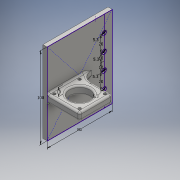
# Autodesk Inventor part: Motor pulley holder
Saved by Autodesk Inventor 2016 (Build 200138000, 138)
## iProperties
Created: 2016-03-20
Part Number: Motor pulley holder
Material: Generic
Document SubType Name: Modeling
Designer: Solomon
Density: 1 g/cm^3
Appearance: Default
Author: Solomon
Autodesk Inventor part; units mm, degrees
ref_plane "YZ Plane" through (0, 0, 0) normal (1, 0, 0) x (0, 1, 0)
ref_plane "XZ Plane" through (0, 0, 0) normal (0, 1, 0) x (-1, 0, 0)
ref_plane "XY Plane" through (0, 0, 0) normal (0, 0, 1) x (1, 0, 0)
sketch "Sketch2" plane through (0, 0, 0) normal (1, 0, 0) x (0, 1, 0)
  line L0 (40, 50) -> (-40, 50)
  line L1 (-40, 50) -> (-40, -50)
  line L2 (-40, -50) -> (40, -50)
  line L3 (40, -50) -> (40, 50)
  line L4 (40, 50) -> (-40, -50) construction
  line L5 (-40, 50) -> (40, -50) construction
  line L6 (40, 50) -> (0, 50)
  line L7 (20, 50) -> (40, 50)
  line L8 (30, 50) -> (30, -50)
  line L9 (30, 0) -> (30, -10)
  line L10 (30, 0) -> (30, 10)
  line L11 (30, -10) -> (30, -30)
  line L12 (30, 10) -> (30, 11.3119)
  line L13 (30, 10) -> (30, 30)
  circle A0 centre (30, -10) radius 2.65
  circle A1 centre (30, 10) radius 2.65
  circle A2 centre (30, 30) radius 2.65
  circle A3 centre (30, -30) radius 2.65
  line L14 (0, 0) -> (-40, 0)
  line L15 (-20, 0) -> (-20, -10)
  line L16 (0, 0) -> (-40, 0)
  line L17 (-40, 0) -> (-40, -10)
  line L18 (-40, -10) -> (0, -10)
  line L19 (0, -10) -> (0, 0)
  line L20 (0, 0) -> (-40, -10) construction
  line L21 (-40, 0) -> (0, -10) construction
  point P0 (-20, -5)
  dimension "d12" = 80
  dimension "d13" = 100
  dimension "d14" = 10
  dimension "d15" = 10
  dimension "d16" = 20
  dimension "d17" = 20
  dimension "d18" = 5.3
  dimension "d19" = 5.3
  dimension "d20" = 5.3
  dimension "d21" = 5.3
  dimension "d22" = 10
  constraints: 44 end point, 11 midpoint, 7 point on line, 4 centre point, 4 coincident, 4 parallel, 3 perpendicular, 2 horizontal, 1 collinear, 1 vertical
  measures "d12" distance of L2.end L1.end
  measures "d13" distance of L1.end L0.end
  measures "d14" distance of L9.start L9.end
  measures "d15" distance of L9.start L10.end
  measures "d16" distance of L9.end L11.end
  measures "d17" distance of L10.end L13.end
  measures "d18" diameter of A0
  measures "d19" diameter of A1
  measures "d20" diameter of A2
  measures "d21" diameter of A3
  measures "d22" distance of L15.start L15.end
extrude "Extrusion2" add sketch "Sketch2" against normal blind 5 contours L3 L2 L8 A3 A0 A1 A2 L0 | L8 A2 A1 A0 A3 L2 L1 L18 L19 L14 L0 | A2 L8 | L8 A2 | A3 L8 | L8 A3 | A1 L8 | L8 A1 | A0 L8 | L8 A0
extrude "Extrusion3" cut sketch "Sketch2" along normal mid plane 24.75 contours A2 L8 | L8 A2 | A3 L8 | L8 A3 | A1 L8 | L8 A1 | A0 L8 | L8 A0
extrude "Extrusion4" add sketch "Sketch2" along normal blind 40 and the other way blind 5 contours L1 L14 L15 L18 | L15 L14 L19 L18
sketch "Sketch3" plane through (0, -40, 0) normal (0, 0, 1) x (1, 0, 0)
  line L0 (40, 0) -> (40, 40) projected
  line L1 (40, 40) -> (0, 40)
  line L2 (0, 40) -> (0, 0)
  line L3 (0, 0) -> (40, 0)
  line L4 (40, 0) -> (40, 40)
  line L5 (35.5, 35.5) -> (4.5, 35.5)
  line L6 (4.5, 35.5) -> (4.5, 4.5)
  line L7 (4.5, 4.5) -> (35.5, 4.5)
  line L8 (35.5, 4.5) -> (35.5, 35.5)
  line L9 (35.5, 35.5) -> (4.5, 4.5) construction
  line L10 (4.5, 35.5) -> (35.5, 4.5) construction
  circle A0 centre (35.5, 35.5) radius 1.65
  circle A1 centre (35.5, 4.5) radius 1.65
  circle A2 centre (4.5, 35.5) radius 1.65
  circle A3 centre (4.5, 4.5) radius 1.65
  point P0 (20, 20)
  dimension "d33" = 31
  dimension "d34" = 31
  dimension "d35" = 3.3
  dimension "d36" = 3.3
  dimension "d37" = 3.3
  dimension "d38" = 3.3
  dimension "d39" = 4.5
  dimension "d40" = 40
  dimension "d41" = 4.5
  dimension "d42" = 40
  constraints: 20 end point, 4 centre point, 4 coincident, 4 parallel, 2 horizontal, 2 midpoint, 2 perpendicular
  measures "d33" distance of L7.end L6.end
  measures "d34" distance of L6.end L5.end
  measures "d35" diameter of A0
  measures "d36" diameter of A1
  measures "d37" diameter of A2
  measures "d38" diameter of A3
  measures "d39" distance between parallel lines of L0 L8
  measures "d40" distance between parallel lines of L0 L2
  measures "d41" distance between parallel lines of L1 L5
  measures "d42" distance between parallel lines of L3 L1
extrude "Extrusion5" cut sketch "Sketch3" along normal mid plane 35.5 contours A2 L6 L5 | L5 L6 A2 | A0 L8 L5 | L5 L8 A0 | A3 L7 L6 | L6 L7 A3 | A1 L7 L8 | L8 L7 A1
sketch "Sketch4" plane through (0, -40, 0) normal (0, 0, 1) x (1, 0, 0)
  line L0 (0, 40) -> (40, 40) projected
  line L1 (0, 0) -> (-5, 0) projected
  line L2 (40, 40) -> (0, 40)
  line L3 (0, 40) -> (0, 0)
  line L4 (0, 0) -> (40, 0)
  line L5 (40, 0) -> (40, 40)
  circle A0 centre (20, 20) radius 12.5
  dimension "d45" = 25
  constraints: 8 end point, 2 parallel, 1 centre point, 1 horizontal, 1 perpendicular
  measures "d45" diameter of A0
extrude "Extrusion6" cut sketch "Sketch4" against normal blind 93.75 contours A0
fillet "Fillet1" radius 15 1 edges at (0, 0, -5)
fillet "Fillet2" radius 2.5 2 edges at (27.5, 0, 0) (4.3934, 4.3934, 0)
fillet "Fillet3" radius 2.5 2 edges at (4.3934, 4.3934, -10) (27.5, 0, -10)
fillet "Fillet4" radius 2.5 5 edges at (40, -0.7322, -0.7322) (40, -21.25, 0) (40, -0.7322, -9.2678) (40, -21.25, -10) (40, 0, -5)
fillet "Fillet5" radius 2.5 5 edges at (39.2678, -40, -0.7322) (40, -40, -5) (39.2678, -40, -9.2678) (18.75, -40, -10) (18.75, -40, 0)
fillet "Fillet6" radius 2 3 edges at (0, 10.3244, -0.7529) (0, -39.2678, -0.7322) (0, -15.7569, 0)
fillet "Fillet7" radius 2 3 edges at (0, -39.2678, -9.2678) (0, 10.5726, -9.1702) (0, -15.7569, -10)
fillet "Fillet8" radius 2 2 edges at (7.5, -20, -10) (7.5, -20, 0)
body "Solid1"
